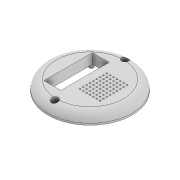
# Autodesk Inventor part: OrTak_lod
Saved by Autodesk Inventor 2022 (Build 260153000, 153)
## iProperties
Created: 2023-02-07
Part Number: OrTak_lod
Material: Generic
Document SubType Name: Modeling
Designer: MVeszpremi
Density: 1 g/cm^3
Appearance: Default
Author: MVeszpremi
Autodesk Inventor part; units mm, degrees
ref_plane "YZ Plane" through (0, 0, 0) normal (1, 0, 0) x (0, 1, 0)
ref_plane "XZ Plane" through (0, 0, 0) normal (0, 1, 0) x (-1, 0, 0)
ref_plane "XY Plane" through (0, 0, 0) normal (0, 0, 1) x (1, 0, 0)
sketch "Sketch1" plane through (0, 0, 0) normal (0, 1, 0) x (-1, 0, 0)
  point P0 (0, 0)
sketch "Sketch2" plane through (0, 0, 0) normal (0, 1, 0) x (-1, 0, 0)
  circle A0 centre (0, 0) radius 62.5
  line L0 (32.5, 35.9442) -> (7.5, 35.9442)
  line L1 (7.5, 35.9442) -> (7.5, -36.0558)
  line L2 (7.5, -36.0558) -> (32.5, -36.0558)
  line L3 (32.5, -36.0558) -> (32.5, 35.9442)
  line L4 (32.5, 35.9442) -> (7.5, -36.0558) construction
  line L5 (7.5, 35.9442) -> (32.5, -36.0558) construction
  line L6 (-5, 19.9442) -> (-35, 19.9442)
  line L7 (-35, 19.9442) -> (-35, -20.0558)
  line L8 (-35, -20.0558) -> (-5, -20.0558)
  line L9 (-5, -20.0558) -> (-5, 19.9442)
  line L10 (-5, 19.9442) -> (-35, -20.0558) construction
  line L11 (-35, 19.9442) -> (-5, -20.0558) construction
  circle A1 centre (-5, 19.9442) radius 1
  circle A2 centre (-5, 14.9442) radius 1
  circle A3 centre (-5, 9.9442) radius 1
  circle A4 centre (-5, 4.9442) radius 1
  circle A5 centre (-5, -0.0558) radius 1
  circle A6 centre (-5, -5.0558) radius 1
  circle A7 centre (-5, -10.0558) radius 1
  circle A8 centre (-5, -15.0558) radius 1
  circle A9 centre (-5, -20.0558) radius 1
  circle A10 centre (-10, 4.9442) radius 1
  circle A11 centre (-10, -0.0558) radius 1
  circle A12 centre (-10, -5.0558) radius 1
  circle A13 centre (-10, -10.0558) radius 1
  circle A14 centre (-10, -15.0558) radius 1
  circle A15 centre (-10, -20.0558) radius 1
  circle A16 centre (-10, 9.9442) radius 1
  circle A17 centre (-10, 19.9442) radius 1
  line L12 (-10, -20.0558) -> (-10, 19.9442)
  circle A18 centre (-10, 14.9442) radius 1
  circle A19 centre (-15, 4.9442) radius 1
  circle A20 centre (-15, -0.0558) radius 1
  circle A21 centre (-15, -5.0558) radius 1
  circle A22 centre (-15, -10.0558) radius 1
  circle A23 centre (-15, -15.0558) radius 1
  circle A24 centre (-15, -20.0558) radius 1
  circle A25 centre (-15, 9.9442) radius 1
  circle A26 centre (-15, 19.9442) radius 1
  line L13 (-15, -20.0558) -> (-15, 19.9442)
  circle A27 centre (-15, 14.9442) radius 1
  circle A28 centre (-20, 4.9442) radius 1
  circle A29 centre (-20, -0.0558) radius 1
  circle A30 centre (-20, -5.0558) radius 1
  circle A31 centre (-20, -10.0558) radius 1
  circle A32 centre (-20, -15.0558) radius 1
  circle A33 centre (-20, -20.0558) radius 1
  circle A34 centre (-20, 9.9442) radius 1
  circle A35 centre (-20, 19.9442) radius 1
  line L14 (-20, -20.0558) -> (-20, 19.9442)
  circle A36 centre (-20, 14.9442) radius 1
  circle A37 centre (-25, 4.9442) radius 1
  circle A38 centre (-25, -0.0558) radius 1
  circle A39 centre (-25, -5.0558) radius 1
  circle A40 centre (-25, -10.0558) radius 1
  circle A41 centre (-25, -15.0558) radius 1
  circle A42 centre (-25, -20.0558) radius 1
  circle A43 centre (-25, 9.9442) radius 1
  circle A44 centre (-25, 19.9442) radius 1
  line L15 (-25, -20.0558) -> (-25, 19.9442)
  circle A45 centre (-25, 14.9442) radius 1
  circle A46 centre (-30, 4.9442) radius 1
  circle A47 centre (-30, -0.0558) radius 1
  circle A48 centre (-30, -5.0558) radius 1
  circle A49 centre (-30, -10.0558) radius 1
  circle A50 centre (-30, -15.0558) radius 1
  circle A51 centre (-30, -20.0558) radius 1
  circle A52 centre (-30, 9.9442) radius 1
  circle A53 centre (-30, 19.9442) radius 1
  line L16 (-30, -20.0558) -> (-30, 19.9442)
  circle A54 centre (-30, 14.9442) radius 1
  circle A55 centre (-35, 4.9442) radius 1
  circle A56 centre (-35, -0.0558) radius 1
  circle A57 centre (-35, -5.0558) radius 1
  circle A58 centre (-35, -10.0558) radius 1
  circle A59 centre (-35, -15.0558) radius 1
  circle A60 centre (-35, -20.0558) radius 1
  circle A61 centre (-35, 9.9442) radius 1
  circle A62 centre (-35, 19.9442) radius 1
  line L17 (-35, -20.0558) -> (-35, 19.9442)
  circle A63 centre (-35, 14.9442) radius 1
  point P0 (20, -0.0558)
  point P1 (-20, -0.0558)
  dimension "d0" = 125
  dimension "d1" = 72
  dimension "d2" = 25
  dimension "d3" = 20
  dimension "d4" = 40
  dimension "d5" = 30
  dimension "d6" = 20
  dimension "d7" = 2
  dimension "d10" = 5
  dimension "d20" = 5
  constraints: 64 centre point, 36 end point, 8 coincident, 4 midpoint, 4 parallel, 3 horizontal, 2 perpendicular, 1 vertical, 142 other
  measures "d0" diameter of A0
  measures "d1" distance of L2.end L0.start
  measures "d2" distance of L0.start L0.end
  measures "d3" horizontal distance of point (0, 0) point (20, -0.056)
  measures "d4" distance of L8.end L6.start
  measures "d5" distance of L7.end L8.end
  measures "d6" horizontal distance of point (0, 0) point (-20, -0.056)
  measures "d7" diameter of A1
  measures "d10" distance of A1.centre A2.centre
  measures "d20" distance of A4.centre A10.centre
extrude "Extrusion1" add sketch "Sketch2" along normal blind 15 contours A0 | L6 A1 L9 A2 A3 A4 A5 A6 A7 A8 A9 L8 A15 L12 A14 A13 A12 A11 A10 A16 A18 A17 | A17 L12 A18 A16 A10 A11 A12 A13 A14 A15 L8 A24 L13 A23 A22 A21 A20 A19 A25 A27 A26 L6 | A26 L13 A27 A25 A19 A20 A21 A22 A23 A24 L8 A33 L14 A32 A31 A30 A29 A28 A34 A36 A35 L6 | A35 L14 A36 A34 A28 A29 A30 A31 A32 A33 L8 A42 L15 A41 A40 A39 A38 A37 A43 A45 A44 L6 | A44 L15 A45 A43 A37 A38 A39 A40 A41 A42 L8 A51 L16 A50 A49 A48 A47 A46 A52 A54 A53 L6 | A53 L16 A54 A52 A46 A47 A48 A49 A50 A51 L8 A60 L7 A59 A58 A57 A56 A55 A61 A63 A62 L6
sketch "Sketch3" plane through (0, 0, 0) normal (0, -1, 0) x (1, 0, 0)
  line L0 (-32.5, 35.9442) -> (-32.5, -36.0558) projected
  line L1 (-7.5, -36.0558) -> (-7.5, 35.9442) projected
  line L2 (-32.5, -36.0558) -> (-7.5, 35.9442)
  line L3 (-7.5, 35.9442) -> (-32.5, 35.9442) projected
  line L4 (-7.5, -36.0558) -> (-32.5, 35.9442)
  line L5 (-35.5, -37.5558) -> (-4.5, -37.5558)
  line L6 (-4.5, -37.5558) -> (-4.5, 37.4442)
  line L7 (-4.5, 37.4442) -> (-35.5, 37.4442)
  line L8 (-35.5, 37.4442) -> (-35.5, -37.5558)
  line L9 (-35.5, -37.5558) -> (-4.5, 37.4442) construction
  line L10 (-4.5, -37.5558) -> (-35.5, 37.4442) construction
  circle A0 centre (-35.5, -37.5558) radius 3
  circle A1 centre (-4.5, 37.4442) radius 3
  circle A2 centre (-4.5, -37.5558) radius 3
  circle A3 centre (-35.5, 37.4442) radius 3
  circle A4 centre (-35.5, -37.5558) radius 1.5
  circle A5 centre (-35.5, 37.4442) radius 1.5
  circle A6 centre (-4.5, 37.4442) radius 1.5
  circle A7 centre (-4.5, -37.5558) radius 1.5
  point P0 (0, 0)
  point P1 (-20, -0.0558)
  dimension "d24" = 75
  dimension "d25" = 31
  dimension "d26" = 6
  dimension "d27" = 6
  dimension "d28" = 6
  dimension "d29" = 6
  dimension "d30" = 3
  dimension "d31" = 3
  dimension "d32" = 3
  dimension "d33" = 3
  constraints: 16 end point, 8 centre point, 8 coincident, 3 midpoint, 2 parallel, 1 horizontal, 1 perpendicular
  measures "d24" distance of L7.end L5.start
  measures "d25" distance of L5.start L5.end
  measures "d26" diameter of A0
  measures "d27" diameter of A1
  measures "d28" diameter of A3
  measures "d29" diameter of A2
  measures "d30" diameter of A4
  measures "d31" diameter of A5
  measures "d32" diameter of A6
  measures "d33" diameter of A7
extrude "Extrusion2" add sketch "Sketch3" along normal blind 5.5 contours A4 L8 A0 L5 | L5 A0 L8 A4 | A2 L6 A7 L5 | L5 A7 L6 A2 | A3 L7 A5 L8 | L8 A5 L7 A3 | A1 L7 A6 L6 | L6 A6 L7 A1
sketch "Sketch4" plane through (0, 0, 0) normal (0, -1, 0) x (1, 0, 0)
  line L0 (10, -30.5) -> (30, -30.5)
  line L1 (30, -30.5) -> (30, -24.5)
  line L2 (30, -24.5) -> (10, -24.5)
  line L3 (10, -24.5) -> (10, -30.5)
  line L4 (10, -30.5) -> (30, -24.5) construction
  line L5 (30, -30.5) -> (10, -24.5) construction
  line L6 (20, -27.5) -> (20, 27.5)
  line L7 (30, 24.5) -> (10, 24.5)
  line L8 (10, 24.5) -> (10, 30.5)
  line L9 (10, 30.5) -> (30, 30.5)
  line L10 (30, 30.5) -> (30, 24.5)
  line L11 (30, 24.5) -> (10, 30.5) construction
  line L12 (10, 24.5) -> (30, 30.5) construction
  point P0 (0, 0)
  point P1 (10, 25.0326)
  dimension "d36" = 6
  dimension "d37" = 20
  dimension "d39" = 27.5
  dimension "d40" = 27.5
  dimension "d41" = 20
  dimension "d47" = 6
  dimension "d48" = 20
  constraints: 26 end point, 4 midpoint, 4 parallel, 2 horizontal, 2 perpendicular, 1 point on line, 1 vertical
  measures "d36" distance of L2.end L0.start
  measures "d37" distance of L0.start L0.end
  measures "d39" vertical distance of L6.end point (0, 0)
  measures "d40" vertical distance of point (0, 0) L6.start
  measures "d41" distance from line of point (0, 0) L6
  measures "d47" distance of L7.end L8.end
  measures "d48" distance of L8.end L9.end
extrude "Extrusion3" add sketch "Sketch4" along normal blind 12.5
sketch "Sketch5" plane through (10, 0, 30.5) normal (0, 0, 1) x (1, 0, 0)
  line L0 (16.2941, -10.1475) -> (3.7941, -10.1475)
  line L1 (3.7941, -10.1475) -> (3.7941, -2.2125)
  line L2 (3.7941, -2.2125) -> (16.2941, -2.2125)
  line L3 (16.2941, -2.2125) -> (16.2941, -10.1475)
  line L4 (16.2941, -10.1475) -> (3.7941, -2.2125) construction
  line L5 (3.7941, -10.1475) -> (16.2941, -2.2125) construction
  point P0 (-10, 0)
  point P1 (10.0441, -6.18)
  dimension "d44" = 12.5
  constraints: 12 end point, 2 midpoint, 2 parallel, 1 horizontal, 1 perpendicular
  measures "d44" distance of L0.start L0.end
extrude "Extrusion4" cut sketch "Sketch5" against normal blind 97
sketch "Sketch6" plane through (0, 0, 0) normal (0, -1, 0) x (1, 0, 0)
  line L0 (0, 0) -> (0, -52)
  circle A0 centre (0, -52) radius 1.5
  line L1 (0, 0) -> (-13.6489, 0)
  circle A1 centre (0, 52) radius 1.5
  dimension "d49" = 52
  dimension "d50" = 3
  constraints: 4 end point, 2 centre point, 1 coincident, 1 horizontal, 1 symmetric about line, 1 vertical, 1 other
  measures "d49" distance of L0.start L0.end
  measures "d50" diameter of A0
extrude "Extrusion5" cut sketch "Sketch6" against normal blind 15
fillet "Fillet1" radius 12.5 1 edges at (62.5, 15, 0)
sketch "Sketch7" plane through (0, 15, 0) normal (0, 1, 0) x (1, 0, 0)
  circle A0 centre (0, -52) radius 1.5 projected
  circle A1 centre (0, -52) radius 5
  circle A2 centre (0, 52) radius 1.5 projected
  circle A3 centre (0, 52) radius 5
  point P0 (0, 0)
  dimension "d54" = 10
  dimension "d55" = 10
  constraints: 2 centre point, 2 coincident
  measures "d54" diameter of A1
  measures "d55" diameter of A3
extrude "Extrusion6" cut sketch "Sketch7" against normal blind 7.5
sketch "Sketch8" plane through (0, 0, 0) normal (0, -1, 0) x (1, 0, 0)
  line L0 (40, 23.1872) -> (0, 23.1872)
  line L1 (0, 23.1872) -> (0, -23.2988)
  line L2 (0, -23.2988) -> (40, -23.2988)
  line L3 (40, -23.2988) -> (40, 23.1872)
  circle A0 centre (20, -0.0558) radius 1 projected
  line L4 (40, 23.1872) -> (0, -23.2988) construction
  line L5 (0, 23.1872) -> (40, -23.2988) construction
  line L6 (-55.2071, -18.94) -> (-39.4239, -18.94)
  line L7 (-39.4239, -18.94) -> (-39.4239, 18.8283)
  line L8 (-39.4239, 18.8283) -> (-55.2071, 18.8283)
  line L9 (-55.2071, 18.8283) -> (-55.2071, -18.94)
  line L10 (-55.2071, -18.94) -> (-39.4239, 18.8283) construction
  line L11 (-39.4239, -18.94) -> (-55.2071, 18.8283) construction
  point P0 (0, 0)
  point P1 (-47.3155, -0.0558)
  constraints: 24 end point, 4 midpoint, 4 parallel, 2 horizontal, 2 perpendicular
extrude "Extrusion7" cut sketch "Sketch8" against normal blind 7.5
sketch "Sketch9" plane through (0, 0, 0) normal (0, -1, 0) x (1, 0, 0)
  line L0 (1.9721, -46.4569) -> (19.7593, -46.4569)
  line L1 (19.7593, -46.4569) -> (19.7593, -29.8556)
  line L2 (19.7593, -29.8556) -> (1.9721, -29.8556)
  line L3 (1.9721, -29.8556) -> (1.9721, -46.4569)
  line L4 (1.9721, -46.4569) -> (19.7593, -29.8556) construction
  line L5 (19.7593, -46.4569) -> (1.9721, -29.8556) construction
  line L6 (3.3838, 30.8664) -> (19.7593, 30.8664)
  line L7 (19.7593, 30.8664) -> (19.7593, 48.0216)
  line L8 (19.7593, 48.0216) -> (3.3838, 48.0216)
  line L9 (3.3838, 48.0216) -> (3.3838, 30.8664)
  line L10 (3.3838, 30.8664) -> (19.7593, 48.0216) construction
  line L11 (19.7593, 30.8664) -> (3.3838, 48.0216) construction
  point P0 (0, 0)
  point P1 (10.8657, -38.1563)
  point P2 (11.5716, 39.444)
  constraints: 24 end point, 4 midpoint, 4 parallel, 2 horizontal, 2 perpendicular, 1 point on line
extrude "Extrusion8" cut sketch "Sketch9" against normal blind 7.5
body "Solid1"
